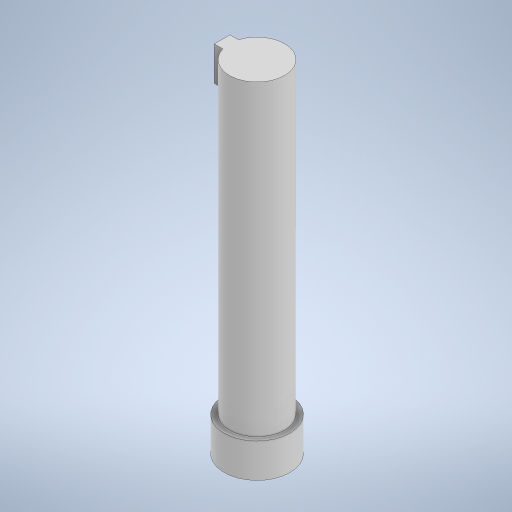
# Autodesk Inventor part: wal_czlon_2
Saved by Autodesk Inventor 2023 (Build 270158000, 158)
## iProperties
Created: 2023-04-09
Part Number: wal_czlon_2
Material: Ogólny
Document SubType Name: Modeling
Designer: Wiktor
Density: 1 g/cm^3
Appearance: Domyślna
Author: Wiktor
Autodesk Inventor part; units mm, degrees
ref_plane "YZ Plane" through (0, 0, 0) normal (1, 0, 0) x (0, 1, 0)
ref_plane "XZ Plane" through (0, 0, 0) normal (0, 1, 0) x (-1, 0, 0)
ref_plane "XY Plane" through (0, 0, 0) normal (0, 0, 1) x (1, 0, 0)
sketch "Szkic1" plane through (0, 0, 0) normal (0, 1, 0) x (-1, 0, 0)
  arc A0 (10.0623, 3) -> (10.0623, -3) centre (0, 0) ccw
  line L0 (13.3003, 3) -> (13.3003, -3)
  line L1 (13.3003, -3) -> (10.0623, -3)
  line L2 (13.3003, 3) -> (10.0623, 3)
  point P0 (13.3003, 0)
  dimension "d0" = 21
  dimension "d1" = 6
  dimension "d2" = 3.238
  constraints: 6 end point, 2 horizontal alignment, 2 point on circle, 1 centre point, 1 coincident, 1 horizontal, 1 midpoint, 1 vertical
  measures "d0" diameter of A0
  measures "d1" distance of L0.start L0.end
  measures "d2" distance of L0.start L2.end
extrude "Wyciągnięcie proste1" add sketch "Szkic1" against normal blind 13
sketch "Szkic3" plane through (0, -13, 0) normal (0, -1, 0) x (1, 0, 0)
  circle A0 centre (0, 0) radius 10.5
  constraints: 1 centre point, 1 coincident
extrude "Wyciągnięcie proste3" add sketch "Szkic3" along normal blind 104
sketch "Szkic4" plane through (0, -117, 0) normal (0, -1, 0) x (1, 0, 0)
  circle A0 centre (0, 0) radius 12.5
  dimension "d9" = 25
  constraints: 1 centre point, 1 coincident
  measures "d9" diameter of A0
extrude "Wyciągnięcie proste4" add sketch "Szkic4" along normal blind 13
